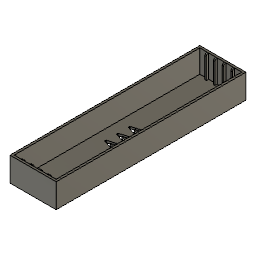
parametric-sh-plate-box (Autodesk Fusion 360 design; units mm, degrees)
Autodesk Fusion 360 part; units mm, degrees
sketch "Skizze1" plane through (0, 0, 0) normal (0, 0, 1) x (1, 0, 0) in component "halfcup"
  line L0 (0, 0) -> (21.3, 0)
  line L1 (21.3, 0) -> (21.3, 87.5)
  line L2 (21.3, 87.5) -> (0, 87.5)
  line L3 (0, 87.5) -> (0, 0)
  line L4 (1, 1) -> (20.3, 1)
  line L5 (20.3, 1) -> (20.3, 86.5)
  line L6 (20.3, 86.5) -> (1, 86.5)
  line L7 (1, 86.5) -> (1, 1)
  line L8 (4.3, 86.5) -> (4.3, 85.5)
  line L9 (4.3, 85.5) -> (5, 85.5)
  line L10 (5, 85.5) -> (5, 86.5)
  dimension "d8" = 87.5
  dimension "d10" = 21.3
  dimension "d11" = 0.7
  dimension "d12" = 1
  dimension "d13" = 3.3
  constraint horizontal L0
  constraint vertical L1
  constraint horizontal L2
  constraint vertical L3
  constraint coincident L0.start L3.end
  constraint coincident L6 L8.start
  constraint perpendicular L6 L8
  constraint perpendicular L8 L9
  constraint coincident L6 L10.end
  constraint perpendicular L6 L10
  measures "d8" distance of L0.start L2.end
  measures "d10" distance of L0.start L0.end
  measures "d11" distance of L8.end L9.end
  measures "d12" distance of L9.end L10.end
  measures "d13" distance of L7 L8
extrude "Extrusion1" add sketch "Skizze1" against normal blind 1 contours L0 L1 L2 L3 | L4 L5 L6 L7 L8 L9 L10 | L6 L8 L9 L10 in component "halfcup"
extrude "Extrusion2" add sketch "Skizze1" along normal blind 10.5 in component "halfcup"
extrude "Extrusion3" add sketch "Skizze1" along normal blind 10.5 contours L6 L8 L9 L10 in component "halfcup"
fillet "Abrundung1" radius 0.9 1 edges at (4.65, 85.5, 10.5) in component "halfcup"
ref_plane "Arbeitsebene1" through (10.65, 43.75, 5.25) normal (0, -1, 0) x (1, 0, 0) in component "halfcup"
pattern_path "Pfadanordnung2" count 4 spacing 4 from (1, 86.5, 10.5) along 1 edges at (12.65, 86.5, 10.5) of "Extrusion3", "Abrundung1" in component "halfcup"
mirror "Spiegeln3" about plane through (10.65, 43.75, 5.25) normal (0, -1, 0) of "Extrusion3", "Abrundung1", "Pfadanordnung2" in component "halfcup"
ref_plane "Arbeitsebene1" through (10.65, 43.75, 4.75) normal (-1, 0, 0) x (0, 1, 0)
ref_plane "Arbeitsebene2" through (10.65, 43.75, 4.75) normal (0, -1, 0) x (-1, 0, 0)
sketch "Skizze1 (2)" plane through (0, 0, 0) normal (0, 0, 1) x (-1, 0, 0)
  line L0 (-17, -2) -> (-17, -1)
  line L1 (-17, -1) -> (-20.3, -1)
  line L2 (-20.3, -1) -> (-20.3, -86.5)
  line L3 (-20.3, -86.5) -> (-17, -86.5)
  line L4 (-17, -86.5) -> (-17, -85.5)
  line L5 (-17, -85.5) -> (-16.3, -85.5)
  line L6 (-16.3, -85.5) -> (-16.3, -86.5)
  line L7 (-16.3, -86.5) -> (-13, -86.5)
  line L8 (-13, -86.5) -> (-13, -85.5)
  line L9 (-13, -85.5) -> (-12.3, -85.5)
  line L10 (-12.3, -85.5) -> (-12.3, -86.5)
  line L11 (-12.3, -86.5) -> (-9, -86.5)
  line L12 (-9, -86.5) -> (-9, -85.5)
  line L13 (-9, -85.5) -> (-8.3, -85.5)
  line L14 (-8.3, -85.5) -> (-8.3, -86.5)
  line L15 (-8.3, -86.5) -> (-5, -86.5)
  line L16 (-5, -86.5) -> (-5, -85.5)
  line L17 (-5, -85.5) -> (-4.3, -85.5)
  line L18 (-4.3, -85.5) -> (-4.3, -86.5)
  line L19 (-4.3, -86.5) -> (-1, -86.5)
  line L20 (-1, -86.5) -> (-1, -1)
  line L21 (-1, -1) -> (-4.3, -1)
  line L22 (-4.3, -1) -> (-4.3, -2)
  line L23 (-4.3, -2) -> (-5, -2)
  line L24 (-5, -2) -> (-5, -1)
  line L25 (-5, -1) -> (-8.3, -1)
  line L26 (-8.3, -1) -> (-8.3, -2)
  line L27 (-8.3, -2) -> (-9, -2)
  line L28 (-9, -2) -> (-9, -1)
  line L29 (-9, -1) -> (-12.3, -1)
  line L30 (-12.3, -1) -> (-12.3, -2)
  line L31 (-12.3, -2) -> (-13, -2)
  line L32 (-13, -2) -> (-13, -1)
  line L33 (-13, -1) -> (-16.3, -1)
  line L34 (-16.3, -1) -> (-16.3, -2)
  line L35 (-16.3, -2) -> (-17, -2)
  spline S0 degree 3 poles (-5.6291, -49.242) (-5.6291, -49.3548) (-5.6823, -49.5009) (-5.7486, -49.5607) knots 0 0 0 0 1 1 1 1
  spline S1 degree 3 poles (-5.7486, -49.5607) (-5.815, -49.6204) (-6.6914, -49.9059) (-7.6873, -50.2047) knots 0 0 0 0 1 1 1 1
  spline S2 degree 3 poles (-7.6873, -50.2047) (-8.6832, -50.5034) (-9.6459, -50.7889) (-9.8318, -50.842) knots 0 0 0 0 1 1 1 1
  spline S3 degree 3 poles (-9.8318, -50.842) (-10.1571, -50.9416) (-10.1571, -50.9416) (-10.1571, -53.5841) knots 0 0 0 0 1 1 1 1
  spline S4 degree 3 poles (-10.1571, -53.5841) (-10.1571, -56.0406) (-10.1704, -56.2331) (-10.2899, -56.3792) knots 0 0 0 0 1 1 1 1
  spline S5 degree 3 poles (-10.2899, -56.3792) (-10.3762, -56.4854) (-10.4891, -56.5385) (-10.6484, -56.5385) knots 0 0 0 0 1 1 1 1
  spline S6 degree 3 poles (-10.6484, -56.5385) (-10.8078, -56.5385) (-10.9206, -56.4854) (-11.0069, -56.3792) knots 0 0 0 0 1 1 1 1
  spline S7 degree 3 poles (-11.0069, -56.3792) (-11.1264, -56.2331) (-11.1331, -56.0406) (-11.1331, -53.3849) knots 0 0 0 0 1 1 1 1
  spline S8 degree 3 poles (-11.1331, -53.3849) (-11.1331, -51.247) (-11.1132, -50.5101) (-11.0468, -50.3839) knots 0 0 0 0 1 1 1 1
  spline S9 degree 3 poles (-11.0468, -50.3839) (-10.9671, -50.2312) (-10.7679, -50.1516) (-9.5662, -49.7864) knots 0 0 0 0 1 1 1 1
  spline S10 degree 3 poles (-9.5662, -49.7864) (-8.8027, -49.554) (-8.0657, -49.3349) (-7.933, -49.2951) knots 0 0 0 0 1 1 1 1
  spline S11 degree 3 poles (-7.933, -49.2951) (-7.7205, -49.2353) (-8.0392, -49.1291) (-11.5978, -48.0602) knots 0 0 0 0 1 1 1 1
  spline S12 degree 3 poles (-11.5978, -48.0602) (-14.1008, -47.31) (-15.5216, -46.8518) (-15.5814, -46.7788) knots 0 0 0 0 1 1 1 1
  spline S13 degree 3 poles (-15.5814, -46.7788) (-15.6279, -46.7124) (-15.6677, -46.573) (-15.6677, -46.4734) knots 0 0 0 0 1 1 1 1
  spline S14 degree 3 poles (-15.6677, -46.4734) (-15.6677, -46.3738) (-15.6079, -46.2344) (-15.5349, -46.168) knots 0 0 0 0 1 1 1 1
  spline S15 degree 3 poles (-15.5349, -46.168) (-15.4619, -46.1016) (-13.6826, -45.5306) (-11.5846, -44.8999) knots 0 0 0 0 1 1 1 1
  spline S16 degree 3 poles (-11.5846, -44.8999) (-9.4866, -44.2758) (-7.7471, -43.758) (-7.7271, -43.7513) knots 0 0 0 0 1 1 1 1
  spline S17 degree 3 poles (-7.7271, -43.7513) (-7.7072, -43.7513) (-9.4334, -43.2202) (-11.5713, -42.5828) knots 0 0 0 0 1 1 1 1
  spline S18 degree 3 poles (-11.5713, -42.5828) (-13.7025, -41.9388) (-15.5017, -41.3678) (-15.5615, -41.3213) knots 0 0 0 0 1 1 1 1
  spline S19 degree 3 poles (-15.5615, -41.3213) (-15.6212, -41.2682) (-15.6677, -41.1288) (-15.6677, -41.0093) knots 0 0 0 0 1 1 1 1
  spline S20 degree 3 poles (-15.6677, -41.0093) (-15.6677, -40.8832) (-15.6146, -40.7305) (-15.5482, -40.6707) knots 0 0 0 0 1 1 1 1
  spline S21 degree 3 poles (-15.5482, -40.6707) (-15.4818, -40.6109) (-13.729, -40.0532) (-11.6576, -39.4358) knots 0 0 0 0 1 1 1 1
  spline S22 degree 3 poles (-11.6576, -39.4358) (-9.5861, -38.8117) (-7.8732, -38.2872) (-7.8467, -38.2606) knots 0 0 0 0 1 1 1 1
  spline S23 degree 3 poles (-7.8467, -38.2606) (-7.8135, -38.2341) (-9.5197, -37.6963) (-11.6244, -37.0722) knots 0 0 0 0 1 1 1 1
  spline S24 degree 3 poles (-11.6244, -37.0722) (-13.8751, -36.4017) (-15.5017, -35.8772) (-15.5615, -35.8108) knots 0 0 0 0 1 1 1 1
  spline S25 degree 3 poles (-15.5615, -35.8108) (-15.6212, -35.7444) (-15.6677, -35.5983) (-15.6677, -35.4854) knots 0 0 0 0 1 1 1 1
  spline S26 degree 3 poles (-15.6677, -35.4854) (-15.6677, -35.3726) (-15.6146, -35.2265) (-15.5482, -35.1668) knots 0 0 0 0 1 1 1 1
  spline S27 degree 3 poles (-15.5482, -35.1668) (-15.4818, -35.107) (-14.6054, -34.8215) (-13.6095, -34.5227) knots 0 0 0 0 1 1 1 1
  spline S28 degree 3 poles (-13.6095, -34.5227) (-12.6136, -34.224) (-11.6509, -33.9385) (-11.465, -33.8854) knots 0 0 0 0 1 1 1 1
  spline S29 degree 3 poles (-11.465, -33.8854) (-11.1331, -33.7858) (-11.1331, -33.7858) (-11.1331, -31.1367) knots 0 0 0 0 1 1 1 1
  spline S30 degree 3 poles (-11.1331, -31.1367) (-11.1331, -28.4877) (-11.1331, -28.4877) (-10.9671, -28.315) knots 0 0 0 0 1 1 1 1
  spline S31 degree 3 poles (-10.9671, -28.315) (-10.8742, -28.2221) (-10.7281, -28.1424) (-10.6484, -28.1424) knots 0 0 0 0 1 1 1 1
  spline S32 degree 3 poles (-10.6484, -28.1424) (-10.5687, -28.1424) (-10.4227, -28.2221) (-10.3297, -28.315) knots 0 0 0 0 1 1 1 1
  spline S33 degree 3 poles (-10.3297, -28.315) (-10.1571, -28.4877) (-10.1571, -28.4877) (-10.1638, -31.3293) knots 0 0 0 0 1 1 1 1
  spline S34 degree 3 poles (-10.1638, -31.3293) (-10.1638, -33.4804) (-10.1837, -34.2173) (-10.2501, -34.3435) knots 0 0 0 0 1 1 1 1
  spline S35 degree 3 poles (-10.2501, -34.3435) (-10.3297, -34.4962) (-10.5289, -34.5759) (-11.7306, -34.941) knots 0 0 0 0 1 1 1 1
  spline S36 degree 3 poles (-11.7306, -34.941) (-12.4941, -35.1734) (-13.2311, -35.3925) (-13.3639, -35.4323) knots 0 0 0 0 1 1 1 1
  spline S37 degree 3 poles (-13.3639, -35.4323) (-13.5763, -35.4921) (-13.2576, -35.5983) (-9.699, -36.6672) knots 0 0 0 0 1 1 1 1
  spline S38 degree 3 poles (-9.699, -36.6672) (-7.196, -37.4175) (-5.7752, -37.8756) (-5.7155, -37.9486) knots 0 0 0 0 1 1 1 1
  spline S39 degree 3 poles (-5.7155, -37.9486) (-5.669, -38.015) (-5.6291, -38.1544) (-5.6291, -38.254) knots 0 0 0 0 1 1 1 1
  spline S40 degree 3 poles (-5.6291, -38.254) (-5.6291, -38.3536) (-5.6889, -38.493) (-5.7686, -38.5594) knots 0 0 0 0 1 1 1 1
  spline S41 degree 3 poles (-5.7686, -38.5594) (-5.8416, -38.6324) (-7.5612, -39.1835) (-9.7189, -39.8275) knots 0 0 0 0 1 1 1 1
  spline S42 degree 3 poles (-9.7189, -39.8275) (-11.8169, -40.4582) (-13.5498, -40.9695) (-13.5763, -40.9761) knots 0 0 0 0 1 1 1 1
  spline S43 degree 3 poles (-13.5763, -40.9761) (-13.5962, -40.9761) (-11.8634, -41.5072) (-9.7256, -42.1446) knots 0 0 0 0 1 1 1 1
  spline S44 degree 3 poles (-9.7256, -42.1446) (-7.5944, -42.7886) (-5.7951, -43.3596) (-5.7354, -43.4061) knots 0 0 0 0 1 1 1 1
  spline S45 degree 3 poles (-5.7354, -43.4061) (-5.6756, -43.4592) (-5.6291, -43.5986) (-5.6291, -43.7181) knots 0 0 0 0 1 1 1 1
  spline S46 degree 3 poles (-5.6291, -43.7181) (-5.6291, -43.8443) (-5.6823, -43.997) (-5.7486, -44.0567) knots 0 0 0 0 1 1 1 1
  spline S47 degree 3 poles (-5.7486, -44.0567) (-5.815, -44.1165) (-7.5678, -44.6742) (-9.6393, -45.2916) knots 0 0 0 0 1 1 1 1
  spline S48 degree 3 poles (-9.6393, -45.2916) (-11.7107, -45.9157) (-13.4236, -46.4402) (-13.4502, -46.4668) knots 0 0 0 0 1 1 1 1
  spline S49 degree 3 poles (-13.4502, -46.4668) (-13.4834, -46.4933) (-11.7771, -47.0311) (-9.6724, -47.6552) knots 0 0 0 0 1 1 1 1
  spline S50 degree 3 poles (-9.6724, -47.6552) (-7.4217, -48.3258) (-5.7951, -48.8503) (-5.7354, -48.9167) knots 0 0 0 0 1 1 1 1
  spline S51 degree 3 poles (-5.7354, -48.9167) (-5.6756, -48.983) (-5.6291, -49.1291) (-5.6291, -49.242) knots 0 0 0 0 1 1 1 1
extrude "Extrusion4" cut sketch "Skizze1 (2)" against normal blind 1 contours S0 S1 S2 S3 S4 S5 S6 S7 S8 S9 S10 S11 S12 S13 S14 S15 S16 S17 S18 S19 S20 S21 S22 S23 S24 S25 S26 S27 S28 S29 S30 S31 S32 S33 S34 S35 S36 S37 S38 S39 S40 S41 S42 S43 S44 S45 S46 S47 S48 S49 S50 S51 in component "halfcup"
chamfer "Fase1" distance 0.3 angle 45 4 edges at (21.3, 43.75, -1) (10.65, 0, -1) (0, 43.75, -1) (10.65, 87.5, -1) in component "halfcup"
component "halfcup" placed x (1, 0, 0) y (0, 1, 0) z (0, 0, 1) at (0, 0, 0)
equation "wall_thickness = 1 mm"
equation "cavity_width = 85.5 mm"
equation "cavity_length = 3.3 mm"
equation "pimple_length = 0.7 mm"
equation "pimple_width = wall_thickness"
equation "amount_of_plates = 5"
equation "heigth = 42.5 mm"
equation "d8 = cavity_width + 2 * wall_thickness"
equation "d9 = -wall_thickness"
equation "d10 = amount_of_plates * ( cavity_length + pimple_length ) + 2 * wall_thickness - pimple_length"
equation "d11 = pimple_length"
equation "d12 = pimple_width"
equation "d13 = cavity_length"
equation "d14 = -wall_thickness"
equation "d16 = höhe"
equation "höhe = 10.5 mm"
equation "d29 = wall_thickness - 0.1 mm"
equation "d30 = amount_of_plates - 1"
equation "d31 = cavity_length + pimple_length"
